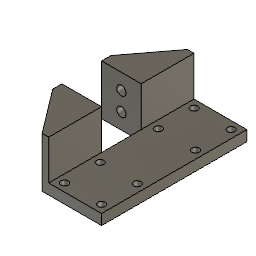
VerbinderLinearfuehrung_Querbalken (Autodesk Fusion 360 design; units mm, degrees)
part number: 2025-10-27-21-09-44-948
Autodesk Fusion 360 part; units mm, degrees
note: some values were not read from the file. Set by a fixed rule: which sketch regions a step uses.
sketch "Skizze1" plane through (0, 0, 0) normal (0, 0, 1) x (1, 0, 0)
  line L0 (0, 0) -> (40, 0)
  line L1 (40, 0) -> (40, 110)
  line L2 (40, 110) -> (0, 110)
  line L3 (0, 110) -> (0, 0)
  dimension "d1" = 40
  dimension "d2" = 110
  constraint horizontal L0
  constraint vertical L1
  constraint horizontal L2
  constraint vertical L3
  constraint coincident L0.start L3.end
  measures "d1" distance of L0.start L0.end
  measures "d2" distance of L0.start L2.end
extrude "Extrusion1" add sketch "Skizze1" along normal blind 9
sketch "Skizze2" plane through (0, 0, 9) normal (0, 0, 1) x (-1, 0, 0)
  line L0 (0, -110) -> (0, 0)
  line L1 (0, 0) -> (-40, 0)
  line L2 (-40, 0) -> (-40, -110)
  line L3 (-40, -110) -> (0, -110)
  line L4 (-40, 0) -> (-35, 0)
  line L5 (-35, 0) -> (-35, -6)
  line L6 (-35, -6) -> (-40, -6)
  line L7 (-40, -6) -> (-40, 0)
  line L8 (0, 0) -> (-6, 0)
  line L9 (-6, 0) -> (-6, -6)
  line L10 (-6, -6) -> (0, -6)
  line L11 (0, -6) -> (0, 0)
  line L12 (0, -110) -> (-6, -110)
  line L13 (-6, -110) -> (-6, -104)
  line L14 (-6, -104) -> (0, -104)
  line L15 (0, -104) -> (0, -110)
  line L16 (-40, -110) -> (-34, -110)
  line L17 (-34, -110) -> (-34, -104)
  line L18 (-34, -104) -> (-40, -104)
  line L19 (-40, -104) -> (-40, -110)
  line L20 (-40, 0) -> (-34, 0)
  line L21 (-34, 0) -> (-34, -6)
  line L22 (-34, -6) -> (-40, -6)
  line L23 (-40, -6) -> (-40, 0)
  line L24 (-40, -110) -> (0, -110)
  line L25 (0, -110) -> (0, -71)
  line L26 (0, -71) -> (-40, -71)
  line L27 (-40, -71) -> (-40, -110)
  line L28 (0, 0) -> (-40, 0)
  line L29 (-40, 0) -> (-40, -39)
  line L30 (-40, -39) -> (0, -39)
  line L31 (0, -39) -> (0, 0)
  line L32 (-40, -39) -> (-34, -39)
  line L33 (-34, -39) -> (-34, -33)
  line L34 (-34, -33) -> (-40, -33)
  line L35 (-40, -33) -> (-40, -39)
  line L36 (0, -39) -> (-6, -39)
  line L37 (-6, -39) -> (-6, -33)
  line L38 (-6, -33) -> (0, -33)
  line L39 (0, -33) -> (0, -39)
  line L40 (0, -71) -> (-6, -71)
  line L41 (-6, -71) -> (-6, -77)
  line L42 (-6, -77) -> (0, -77)
  line L43 (0, -77) -> (0, -71)
  line L44 (-40, -71) -> (-34, -71)
  line L45 (-34, -71) -> (-34, -77)
  line L46 (-34, -77) -> (-40, -77)
  line L47 (-40, -77) -> (-40, -71)
  circle A0 centre (-6, -6) radius 2.75
  circle A1 centre (-34, -6) radius 2.75
  circle A2 centre (-6, -33) radius 2.75
  circle A3 centre (-34, -33) radius 2.75
  circle A4 centre (-34, -77) radius 2.75
  circle A5 centre (-6, -77) radius 2.75
  circle A6 centre (-6, -104) radius 2.75
  circle A7 centre (-34, -104) radius 2.75
  dimension "d5" = 6
  dimension "d6" = 6
  dimension "d7" = 6
  dimension "d8" = 6
  dimension "d9" = 6
  dimension "d10" = 6
  dimension "d11" = 6
  dimension "d12" = 6
  dimension "d13" = 6
  dimension "d14" = 40
  dimension "d15" = 39
  dimension "d16" = 40
  dimension "d17" = 39
  dimension "d18" = 6
  dimension "d19" = 6
  dimension "d20" = 6
  dimension "d21" = 6
  dimension "d22" = 6
  dimension "d23" = 6
  dimension "d24" = 6
  dimension "d25" = 6
  dimension "d26" = 5.5
  dimension "d27" = 5.5
  dimension "d28" = 5.5
  dimension "d29" = 5.5
  dimension "d30" = 5.5
  dimension "d31" = 5.5
  dimension "d32" = 5.5
  dimension "d33" = 5.5
  constraint horizontal L4
  constraint vertical L5
  constraint horizontal L6
  constraint vertical L7
  constraint coincident L1.end L2.start
  constraint horizontal L8
  constraint vertical L9
  constraint horizontal L10
  constraint vertical L11
  constraint coincident L0.end L1.start
  constraint horizontal L12
  constraint vertical L13
  constraint horizontal L14
  constraint vertical L15
  constraint coincident L0.start L3.end
  constraint horizontal L16
  constraint vertical L17
  constraint horizontal L18
  constraint vertical L19
  constraint coincident L2.end L3.start
  constraint horizontal L20
  constraint vertical L21
  constraint horizontal L22
  constraint vertical L23
  constraint horizontal L24
  constraint vertical L25
  constraint horizontal L26
  constraint vertical L27
  constraint horizontal L28
  constraint vertical L29
  constraint horizontal L30
  constraint vertical L31
  constraint horizontal L32
  constraint vertical L33
  constraint horizontal L34
  constraint vertical L35
  constraint horizontal L36
  constraint vertical L37
  constraint horizontal L38
  constraint vertical L39
  constraint horizontal L40
  constraint vertical L41
  constraint horizontal L42
  constraint vertical L43
  constraint horizontal L44
  constraint vertical L45
  constraint horizontal L46
  constraint vertical L47
  constraint coincident L9.end L10.start
  constraint coincident L21.end L22.start
  constraint coincident L37.end L38.start
  constraint coincident L33.end L34.start
  constraint coincident L45.end L46.start
  constraint coincident L41.end L42.start
  constraint coincident L13.end L14.start
  constraint coincident L17.end L18.start
  measures "d5" distance of L1.end L6.end
  measures "d6" distance of L0.end L8.end
  measures "d7" distance of L0.end L10.end
  measures "d8" distance of L0.start L12.end
  measures "d9" distance of L0.start L14.end
  measures "d10" distance of L2.end L16.end
  measures "d11" distance of L2.end L18.end
  measures "d12" distance of L1.end L20.end
  measures "d13" distance of L1.end L6.end
  measures "d14" distance of L2.end L0.start
  measures "d15" distance of L2.end L26.end
  measures "d16" distance of L0.end L1.end
  measures "d17" distance of L0.end L30.end
  measures "d18" distance of L29.end L32.end
  measures "d19" distance of L29.end L34.end
  measures "d20" distance of L30.end L36.end
  measures "d21" distance of L30.end L38.end
  measures "d22" distance of L25.end L40.end
  measures "d23" distance of L25.end L42.end
  measures "d24" distance of L26.end L44.end
  measures "d25" distance of L26.end L46.end
  measures "d26" diameter of A0
  measures "d27" diameter of A1
  measures "d28" diameter of A2
  measures "d29" diameter of A3
  measures "d30" diameter of A4
  measures "d31" diameter of A5
  measures "d32" diameter of A6
  measures "d33" diameter of A7
extrude "Extrusion2" cut sketch "Skizze2" against normal blind 10 contours L13 L14 A6 | L13 L14 A6 | L41 L42 A5 | L41 L42 A5 | L17 L18 A7 | L17 L18 A7 | L37 L38 A2 | L37 L38 A2 | L45 L46 A4 | L45 L46 A4 | L9 L10 A0 | L9 L10 A0 | L33 L34 A3 | L33 L34 A3 | L6 L21 L22 A1 | L5 L21 L22 A1 | L5 L6 L22 A1
extrude "Extrusion11" cut 1 faces at (24.2083, 48.4605, 9) along direction (0, 0, -1) blind 1
sketch "Skizze10" plane through (0, 0, 0) normal (0, 0, 1) x (1, 0, 0)
  line L0 (0, 0) -> (0, 110)
  line L1 (0, 55) -> (0, 40)
  line L2 (0, 40) -> (-30, 40)
  line L3 (-30, 70) -> (0, 70)
  line L4 (0, 70) -> (0, 40)
  line L5 (-30, 70) -> (0, 70)
  line L6 (0, 70) -> (0, 77)
  line L7 (0, 77) -> (-30, 77)
  line L8 (-30, 77) -> (-30, 70)
  line L9 (-30, 40) -> (0, 40)
  line L10 (0, 40) -> (0, 33)
  line L11 (0, 33) -> (-30, 33)
  line L12 (-30, 33) -> (-30, 40)
  line L13 (0, 77) -> (-5, 77)
  line L14 (-5, 77) -> (-5, 110)
  line L15 (-5, 110) -> (0, 110)
  line L16 (0, 110) -> (0, 77)
  line L17 (0, 33) -> (-5, 33)
  line L18 (-5, 33) -> (-5, 0)
  line L19 (-5, 0) -> (0, 0)
  line L20 (0, 0) -> (0, 33)
  dimension "d69" = 15
  dimension "d70" = 30
  dimension "d71" = 30
  dimension "d72" = 7
  dimension "d73" = 7
  constraint coincident L0.start L19.end
  constraint vertical L0
  constraint midpoint L0 L1.start
  constraint parallel L0 L1
  constraint horizontal L2
  constraint horizontal L3
  constraint vertical L4
  constraint horizontal L5
  constraint vertical L6
  constraint horizontal L7
  constraint vertical L8
  constraint coincident L0 L6.end
  constraint horizontal L9
  constraint vertical L10
  constraint horizontal L11
  constraint vertical L12
  constraint coincident L0 L10.end
  constraint horizontal L13
  constraint vertical L14
  constraint horizontal L15
  constraint vertical L16
  constraint horizontal L17
  constraint vertical L18
  constraint horizontal L19
  constraint vertical L20
  measures "d69" distance of L1.start L1.end
  measures "d70" distance of L1.end L2.end
  measures "d71" distance of L1.end L3.end
  measures "d72" distance of L5 L7
  measures "d73" distance of L2 L11
extrude "Extrusion12" add sketch "Skizze10" along normal blind 38
sketch "Skizze11" plane through (0, 0, 0) normal (0, 0, 1) x (1, 0, 0)
  line L0 (-5, 0) -> (-5, 33)
  line L1 (-5, 33) -> (-30, 33)
  line L2 (-30, 33) -> (-5, 0)
  line L3 (-5, 110) -> (-5, 77)
  line L4 (-5, 77) -> (-30, 77)
  line L5 (-5, 110) -> (-30, 77)
  constraint vertical L0
  constraint perpendicular L0 L1
  constraint perpendicular L1 L3
  constraint perpendicular L3 L4
extrude "Extrusion13" add sketch "Skizze11" along normal blind 5
extrude "Extrusion14" add 2 faces at (-13.3333, 88, 5) (-13.3333, 22, 5) along direction (0, 0, 1) blind 5 from surface at 28
sketch "Skizze12" plane through (0, 33, 0) normal (0, -1, 0) x (1, 0, 0)
  line L0 (-5, 33) -> (-30, 33)
  line L1 (-30, 33) -> (-30, 5)
  line L2 (-30, 5) -> (-5, 5)
  line L3 (-5, 5) -> (-5, 33)
  line L4 (-30, 33) -> (-15, 33)
  line L5 (-15, 33) -> (-15, 5)
  line L6 (-15, 33) -> (-15, 26)
  line L7 (-15, 5) -> (-15, 12)
  circle A0 centre (-15, 12) radius 3.5
  circle A1 centre (-15, 26) radius 3.5
  dimension "d81" = 15
  dimension "d82" = 7
  dimension "d83" = 7
  dimension "d84" = 7
  dimension "d85" = 7
  constraint coincident L0.end L1.start
  constraint perpendicular L1 L4
  constraint coincident L2 L5.end
  constraint perpendicular L2 L5
  constraint perpendicular L4 L6
  constraint perpendicular L2 L7
  constraint coincident L7.end A0.centre
  constraint coincident L6.end A1.centre
  measures "d81" distance of L0.end L4.end
  measures "d82" distance of L4.end L6.end
  measures "d83" distance of L5.end L7.end
  measures "d84" diameter of A0
  measures "d85" diameter of A1
extrude "Extrusion15" cut sketch "Skizze12" against normal blind 95 contours L5 L6 A1 | L5 L6 A1 | L5 L7 A0 | L5 L7 A0
